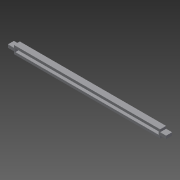
# Autodesk Inventor part: top_cover_side
Saved by Autodesk Inventor 2014 SP1 (Build 180222100, 222)
## iProperties
Created: 2014-02-23
Part Number: top_cover_side
Material: Wood (Birch)
Document SubType Name: Modeling
Designer: Chris
Density: 0.55 g/cm^3
Appearance: Birch - Natural Polished
Mass: 105.197 g
Surface Area: 535.281 cm^2
Volume: 191.268 cm^3
Author: Chris
Autodesk Inventor part; units mm, degrees
ref_plane "YZ Plane" through (0, 0, 0) normal (1, 0, 0) x (0, 1, 0)
ref_plane "XZ Plane" through (0, 0, 0) normal (0, 1, 0) x (-1, 0, 0)
ref_plane "XY Plane" through (0, 0, 0) normal (0, 0, 1) x (1, 0, 0)
sketch "Sketch1" plane through (0, 0, 0) normal (0, 0, 1) x (1, 0, 0)
  line L0 (-47.625, 38.3646) -> (-47.625, 30.4271)
  line L1 (-47.625, 30.4271) -> (-66.675, 30.4271)
  line L2 (-66.675, 30.4271) -> (-66.675, 20.9021)
  line L3 (-66.675, 20.9021) -> (-47.625, 20.9021)
  line L4 (-47.625, 20.9021) -> (-47.625, 12.9646)
  line L5 (-47.625, 38.3646) -> (185.7375, 38.3646)
  line L6 (185.7375, 38.3646) -> (185.7375, 12.9646)
  line L7 (185.7375, 12.9646) -> (-47.625, 12.9646)
  line L8 (-47.625, 12.9646) -> (-47.625, 38.3646)
  line L9 (-47.625, 20.9021) -> (-66.675, 20.9021)
  line L10 (-66.675, 20.9021) -> (-66.675, 30.4271)
  line L11 (-66.675, 30.4271) -> (-47.625, 30.4271)
  line L12 (-47.625, 30.4271) -> (-47.625, 20.9021)
  point P0 (0, 0)
  dimension "d0" = 7.9375
  dimension "d1" = 19.05
  dimension "d2" = 9.525
  dimension "d3" = 7.9375
  dimension "d4" = 25.4
  dimension "d6" = 252.4125
  constraints: 26 end point, 6 perpendicular, 4 parallel, 2 horizontal, 1 vertical
  measures "d0" distance of L0.start L0.end
  measures "d1" distance of L0.end L1.end
  measures "d2" distance of L1.end L2.end
  measures "d3" distance of L3.end L4.end
  measures "d4" distance of L5.end L6.end
  measures "d6" distance between parallel lines of L6 L2
extrude "Extrusion1" add sketch "Sketch1" along normal blind 19.05
mirror "Mirror1" about plane through (185.7375, 12.9646, 0) normal (1, 0, 0) of "Extrusion1"
sketch "Sketch2" plane through (0, 0, 19.05) normal (0, 0, 1) x (1, 0, 0)
  line L0 (-66.675, 30.4271) -> (-66.675, 20.9021) projected
  line L1 (-47.625, 12.9646) -> (419.1, 12.9646) projected
  line L2 (438.15, 30.4271) -> (438.15, 20.9021) projected
  line L3 (-47.625, 38.3646) -> (419.1, 38.3646) projected
  line L4 (-42.8625, 30.4271) -> (414.3375, 30.4271)
  line L5 (414.3375, 30.4271) -> (414.3375, 20.9021)
  line L6 (414.3375, 20.9021) -> (-42.8625, 20.9021)
  line L7 (-42.8625, 20.9021) -> (-42.8625, 30.4271)
  point P0 (0, 0)
  dimension "d10" = 7.9375
  dimension "d11" = 7.9375
  dimension "d12" = 9.525
  dimension "d13" = 23.8125
  dimension "d14" = 23.8125
  constraints: 8 end point, 2 parallel, 1 horizontal, 1 perpendicular
  measures "d10" distance between parallel lines of L3 L4
  measures "d11" distance between parallel lines of L1 L6
  measures "d12" distance between parallel lines of L6 L4
  measures "d13" distance between parallel lines of L0 L7
  measures "d14" distance between parallel lines of L2 L5
extrude "Extrusion2" cut sketch "Sketch2" against normal blind 9.525
equation "\"d11\" = d10"
body "Solid1"
